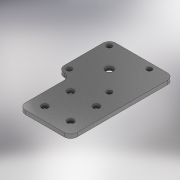
# Autodesk Inventor part: ActuatorPulleyPlate
Saved by Autodesk Inventor 2020.3 (Build 243373000, 373)
## iProperties
Created: 2021-08-04
Part Number: ActuatorPulleyPlate
Material: Aluminum 6061
Document SubType Name: Modeling
Designer: justi
Density: 2.7 g/cm^3
Appearance: Honed - Dark Gray
Author: justi
Autodesk Inventor part; units mm, degrees
ref_plane "YZ Plane" through (0, 0, 0) normal (1, 0, 0) x (0, 1, 0)
ref_plane "XZ Plane" through (0, 0, 0) normal (0, 1, 0) x (-1, 0, 0)
ref_plane "XY Plane" through (0, 0, 0) normal (0, 0, 1) x (1, 0, 0)
sketch "Sketch1" plane through (0, 0, 0) normal (0, 1, 0) x (-1, 0, 0)
  line L0 (25, 40) -> (-25, 40)
  line L1 (-25, 40) -> (-25, -40)
  line L2 (-25, -40) -> (25, -40)
  line L3 (25, -40) -> (25, 40)
  line L4 (25, 40) -> (15, 40)
  line L5 (15, 40) -> (15, 0)
  line L6 (15, 0) -> (25, 0)
  line L7 (25, -40) -> (25, -35.5) construction
  line L8 (25, -35.5) -> (20.5, -35.5) construction
  line L9 (20.5, -35.5) -> (20.5, -4.5) construction
  line L10 (20.5, -4.5) -> (-10.5, -4.5) construction
  line L11 (-10.5, -4.5) -> (-10.5, -35.5) construction
  line L12 (-10.5, -35.5) -> (20.5, -35.5) construction
  circle A0 centre (5, -20) radius 3
  circle A1 centre (20.5, -4.5) radius 2
  circle A2 centre (20.5, -35.5) radius 2
  circle A3 centre (-10.5, -4.5) radius 2
  circle A4 centre (-10.5, -35.5) radius 2
  line L13 (15, 40) -> (5, 40) construction
  line L14 (5, 40) -> (5, 30) construction
  line L15 (5, 30) -> (15, 30) construction
  line L16 (15, 30) -> (15, 40) construction
  line L17 (5, 30) -> (-15, 30) construction
  line L18 (-15, 30) -> (-15, 10) construction
  line L19 (-15, 10) -> (5, 10) construction
  line L20 (5, 10) -> (5, 30) construction
  circle A5 centre (5, 30) radius 2.5
  circle A6 centre (5, 10) radius 2.5
  circle A7 centre (-15, 30) radius 2.5
  circle A8 centre (-15, 10) radius 2.5
  dimension "d0" = 50
  dimension "d1" = 80
  dimension "d2" = 10
  dimension "d3" = 40
  dimension "d4" = 4.5
  dimension "d5" = 4.5
  dimension "d6" = 31
  dimension "d7" = 31
  dimension "d8" = 31
  dimension "d9" = 6
  dimension "d10" = 4
  dimension "d11" = 4
  dimension "d12" = 4
  dimension "d13" = 4
  dimension "d14" = 10
  dimension "d15" = 10
  dimension "d16" = 20
  dimension "d17" = 20
  dimension "d18" = 5
  dimension "d19" = 5
  dimension "d20" = 5
  dimension "d21" = 5
  constraints: 42 end point, 17 coincident, 9 centre point, 8 perpendicular, 6 parallel, 3 horizontal, 2 point on line, 1 midpoint
  measures "d0" distance of L2.end L1.end
  measures "d1" distance of L1.end L0.end
  measures "d2" distance of L0.start L4.end
  measures "d3" distance of L4.end L5.end
  measures "d4" distance of L2.end L7.end
  measures "d5" distance of L7.end L8.end
  measures "d6" distance of L8.end L9.end
  measures "d7" distance of L9.end L10.end
  measures "d8" distance of L10.end L11.end
  measures "d9" diameter of A0
  measures "d10" diameter of A1
  measures "d11" diameter of A2
  measures "d12" diameter of A3
  measures "d13" diameter of A4
  measures "d14" distance of L15.end L14.end
  measures "d15" distance of L14.end L13.end
  measures "d16" distance of L19.end L18.end
  measures "d17" distance of L18.end L17.end
  measures "d18" diameter of A5
  measures "d19" diameter of A6
  measures "d20" diameter of A7
  measures "d21" diameter of A8
extrude "Extrusion1" add sketch "Sketch1" along normal blind 3 contours L5 L6 L3 L2 L1 L0
fillet "Fillet1" radius 5 6 edges at (-15, 1.5, 40) (-25, 1.5, 0) (-25, 1.5, -40) (25, 1.5, 40) (25, 1.5, -40) (-15, 1.5, 0)
body "Solid1"
